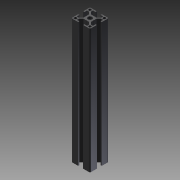
# Autodesk Inventor part: HFS6-3030-200
Saved by Autodesk Inventor 2011 SP1 (Build 150282100, 282)
## iProperties
Created: 2016-11-23
Part Number: HFS6-3030-200
Catalog Web Link: www.cadenas.de
Description: NEFS6-3030, NEFSB6-3030, EFS6-3030, EFSB6-3030, HFS6-3030, HFSB6-3030, CAF6-3030, HFSY6-3030, NFSL6-3030,  HFSL6-3030, HFSLB6-3030, GFS6-3030-HFS6 Series Aluminum Extrusions 30 Square -1 Slot-
Vendor: MISUMI
Document SubType Name: Modeling
Designer: psAdmin
Manufacturer: MISUMI
Mass: 66.3829 g
Surface Area: 634.997 cm^2
Volume: 66.3829 cm^3
Density: 1 g/cm^3
Category: PARTsolutions
Company: MISUMI
Title: HFS6-3030-200
Author: Cadenas PARTsolutions
Comments: HFS6 Series Aluminum Extrusions 30 Square -1 Slot-
PSOL_IDENT_0: {$CADENAS_DATA\23d-libs\misumi\metric\38_al_extrusions_blackets\6\hfs6_3030.prj},609 {VTYP=3D},{NB=H
PSOL_IDENT_1: FS6-3030-200},{LINA=HFS6-3030-200},{NN=NEFS6-3030, NEFSB6-3030, EFS6-3030, EFSB6-3030, HFS6-3030, HF
PSOL_IDENT_2: SB6-3030, CAF6-3030, HFSY6-3030, NFSL6-3030,  HFSL6-3030, HFSLB6-3030, GFS6-3030},{DATE=17.06.2016 0
PSOL_IDENT_3: 5:53:17},{GEOMDATE=28.10.2014 00:00:00},{VERSION=},{LINEID=130},{LINESUBID=-1},{WBVAR=L,ALT1,ALT2,AL
PSOL_IDENT_4: T3,ALT4,ALT5,CP5,DL5,DR5,ALT6,ALT9,ALT10,ALT11,DD6SE,DD6,HP6,NHL6,DL6,NHR6,DR6,ALT7,ALT8,NH9,AH,BH,C
PSOL_IDENT_5: H,DH,EH,NH10,AV,BV,CV,DV,EV,NH11,AP,BP,CP,DP,EP,ALT12,ALT13,Z,NH12,XA,XB,XC,XD,XE,NH13,YA,YB,YC,YD,Y
PSOL_IDENT_6: E,ALT14,HP14,DL14,DR14,ALT15,HP15,DL15,DR15,ALT16,HP16,DL16,DR16,ALT17,HQ17,JLP,ALT19,ALT20}  {NB=HF
PSOL_IDENT_7: S6-3030-200},{LINA=HFS6-3030-200},{KT=DUMMY},{PN=HFS6-3030-200},{TPS=HFS6-3030},{MAT=A6N01SS-T5 Alum
PSOL_IDENT_8: inum Alloy},{ST=Clear Anodize},{FRMW=30},{FRMH=30},{FRD=6.8},{L=200.0},{MASS=0.90},{SA=333},{LX=2.83
PSOL_IDENT_9: x10^4},{LY=2.83x10^4},{ALT1=},{M1=0},{IDM1=6.647},{DALT1=4.2},{DPL1=0},{DPR1=0},{ALT1PN=},{ALT2=},{A
PSOL_IDENT_10: LT2ALG= '','w/o End Tapping (Heli-Coil Insert)','LHP','with LHP (Tapping on the Left (Heli-Coil Inse
PSOL_IDENT_11: rt))','RHP','with RHP (Tapping on the Right (Heli-Coil Insert))','HPW','with HPW (Tapping on Both En
PSOL_IDENT_12: ds (Heli-Coil Insert))' },{M2=0},{DP2=0},{ALT2PN=},{ALT3=},{ALT3ALG= '','w/o Tapping (Corner Section
PSOL_IDENT_13: )','LSP','with LSP (Tapping (Corner Section))','RSP','with RSP (Tapping (Corner Section))','SPW','wi
PSOL_IDENT_14: th SPW (Tapping (Corner Section))' },{M3=0},{IDM3=4.134},{DP3=0},{ALT3PN=},{ALT4=},{ALT4ALG= '', 'w/
PSOL_IDENT_15: o SC (High Precision Cut)', 'SC', 'with SC (High Precision Cut)' },{ALT4PN=},{ALT5=},{ALT5ALG= '','w
PSOL_IDENT_16: /o 45 Degree Cut','1','with 45 Degree Cut' },{CP5=},{CP5ALG= '','N/A' },{DL5=},{DL5ALG= '','N/A' },{
PSOL_IDENT_17: DR5=},{DR5ALG= '','N/A' },{FRMLALT5=0},{FRMRALT5=0},{ALT5PN=},{ALT6=},{ALT6ALG= '','w/o Fastening Lo
PSOL_IDENT_18: cation Wrench Access Hole Alterations','1','with Fastening Location Wrench Access Hole Alterations'
PSOL_IDENT_19: },{ALT9=},{ALT9ALG= '','w/o Location Specified Wrench Access Hole Alteratons (Horizontal)','1','with
PSOL_IDENT_20: Location Specified Wrench Access Hole Alteratons (Horizontal)' },{ALT10=},{ALT10ALG= '','w/o Locati
PSOL_IDENT_21: on Specified Wrench Access Hole Alteratons (Vertical)','1','with Location Specified Wrench Access Ho
PSOL_IDENT_22: le Alteratons (Vertical)' },{ALT11=},{ALT11ALG= '','w/o Location Specified Wrench Access Hole Altera
PSOL_IDENT_23: tons (Crisscross)','1','with Location Specified Wrench Access Hole Alteratons (Crisscross)' },{DD6SE=
PSOL_IDENT_24: },{DD6SEALG= '','N/A' },{DD6=0},{DD6ALG=0},{HP6=},{HP6ALG= '','N/A' },{NHL6=},{NHL6ALG= '','N/A' },{
PSOL_IDENT_25: DL6=},{DL6ALG= '','N/A' },{NHR6=},{NHR6ALG= '','N/A' },{DR6=},{DR6ALG= '','N/A' },{DD6PN=},{HL6=0},{
PSOL_IDENT_26: HL6D=0},{HR6=0},{HR6D=0},{J6=0},{J6D=0},{K6=0},{K6D=0},{ALT7=},{ALT7ALG= '','N/A' },{ALT8=},{ALT8ALG=
PSOL_IDENT_27: '','N/A' },{ALT678PN=},{NH9=0},{NH9MAX=5},{NH9ALG=[0]},{AH=0.0},{AHMIN=7},{AHMAX=195},{AHALG=[0]},{
PSOL_IDENT_28: BH=0.0},{BHMIN=2},{BHMAX=197},{BHALG=[0]},{CH=0.0},{CHMIN=2},{CHMAX=199},{CHALG=[0]},{DH=0.0},{DHMIN=
PSOL_IDENT_29: 2},{DHMAX=201},{DHALG=[0]},{EH=0.0},{EHMIN=2},{EHMAX=193},{EHALG=[0]},{NH10=0},{NH10MAX=5},{NH10ALG=
PSOL_IDENT_30: [0]},{AV=0.0},{AVMIN=7},{AVMAX=195},{AVALG=[0]},{BV=0.0},{BVMIN=2},{BVMAX=197},{BVALG=[0]},{CV=0.0},
PSOL_IDENT_31: {CVMIN=2},{CVMAX=199},{CVALG=[0]},{DV=0.0},{DVMIN=2},{DVMAX=201},{DVALG=[0]},{EV=0.0},{EVMIN=2},{EVM
PSOL_IDENT_32: AX=193},{EVALG=[0]},{NH11=0},{NH11MAX=5},{NH11ALG=[0]},{AP=0.0},{APMIN=7},{APMAX=195},{APALG=[0]},{B
PSOL_IDENT_33: P=0.0},{BPMIN=2},{BPMAX=197},{BPALG=[0]},{CP=0.0},{CPMIN=2},{CPMAX=199},{CPALG=[0]},{DP=0.0},{DPMIN=
PSOL_IDENT_34: 2},{DPMAX=201},{DPALG=[0]},{EP=0.0},{EPMIN=2},{EPMAX=193},{EPALG=[0]},{ALT9PN=},{ALT10PN=},{ALT11PN=
PSOL_IDENT_35: },{ALT91011PN=},{ALT12=},{ALT12ALG= '','w/o Counterbore Hole in Specified Position (Vertical)','1','
PSOL_IDENT_36: with Counterbore Hole in Specified Position (Vertical)' },{ALT13=},{ALT13ALG= '','w/o Counterbore Ho
PSOL_IDENT_37: le in Specified Position (Horizontal)','1','with Counterbore Hole in Specified Position (Horizontal)'
PSOL_IDENT_38: },{Z=},{ZALG= '','N/A' },{DD12=0.0},{DD112=0.0},{NH12=0},{NH12MAX=5},{NH12ALG=[0]},{XA=0.0},{XAMIN=
PSOL_IDENT_39: 7},{XAMAX=195},{XAALG=[0]},{XB=0.0},{XBMIN=2},{XBMAX=197},{XBALG=[0]},{XC=0.0},{XCMIN=2},{XCMAX=199}
PSOL_IDENT_40: ,{XCALG=[0]},{XD=0.0},{XDMIN=2},{XDMAX=201},{XDALG=[0]},{XE=0.0},{XEMIN=2},{XEMAX=193},{XEALG=[0]},{
PSOL_IDENT_41: NH13=0},{NH13MAX=5},{NH13ALG=[0]},{YA=0.0},{YAMIN=7},{YAMAX=195},{YAALG=[0]},{YB=0.0},{YBMIN=2},{YBM
PSOL_IDENT_42: AX=197},{YBALG=[0]},{YC=0.0},{YCMIN=2},{YCMAX=199},{YCALG=[0]},{YD=0.0},{YDMIN=2},{YDMAX=201},{YDALG=
PSOL_IDENT_43: [0]},{YE=0.0},{YEMIN=2},{YEMAX=193},{YEALG=[0]},{ALT12PN=},{ALT13PN=},{ALT1213PN=},{ALT14=},{ALT14AL
PSOL_IDENT_44: G= '','w/o D Type Hole Alteration','1','with D Type Hole Alteration' },{HP14=},{HP14ALG= '','N/A' },
PSOL_IDENT_45: {DL14=},{DL14ALG= '','N/A' },{DR14=},{DR14ALG= '','N/A' },{H14=0},{D14=0.0},{ALT14PN=},{ALT15=},{ALT
PSOL_IDENT_46: 15ALG= '','w/o S Type Hole Alteration','1','with S Type Hole Alteration' },{HP15=},{HP15ALG= '','N/A'
PSOL_IDENT_47: },{DL15=},{DL15ALG= '','N/A' },{DR15=},{DR15ALG= '','N/A' },{H15=0},{D115=0.0},{D215=0.0},{ALT15PN=
PSOL_IDENT_48: },{ALT16=},{ALT16ALG= '','w/o M Type Hole Alteration','1','with M Type Hole Alteration' },{HP16=},{H
PSOL_IDENT_49: P16ALG= '','N/A' },{DL16=},{DL16ALG= '','N/A' },{DR16=},{DR16ALG= '','N/A' },{H116=0},{D16=0.0},{ALT
PSOL_IDENT_50: 16PN=},{ALT17=},{ALT17ALG= '','w/o L Type Hole Alteration (Top)','1','with L Type Hole Alteration (T
PSOL_IDENT_51: op)' },{HQ17=0},{HQ17ALG=0},{JLP=0},{JLPMIN=4.9},{JLPMAX=0},{JLPALG=[0]},{L17=0},{D17=0.0},{ALT17PN=
PSOL_IDENT_52: },{ALT19=},{ALT19ALG= '','N/A' },{M19=0},{DP19=0},{ALT19PN=},{ALT20=},{ALT20PN=},{ERRORALT01=OK},{ER
PSOL_IDENT_53: RORALT02=OK},{ERRORALT03=OK},{ERRORALT05=OK},{ERRORALT06091=OK},{ERRORALT06092=OK},{ERRORALT06093=OK
PSOL_IDENT_54: },{ERRORALT06094=OK},{ERRORALT06101=OK},{ERRORALT06102=OK},{ERRORALT06103=OK},{ERRORALT06104=OK},{ER
PSOL_IDENT_55: RORALT06111=OK},{ERRORALT06112=OK},{ERRORALT06113=OK},{ERRORALT06114=OK},{ERRORALT06121=OK},{ERRORAL
PSOL_IDENT_56: T06122=OK},{ERRORALT06123=OK},{ERRORALT06124=OK},{ERRORALT06131=OK},{ERRORALT06132=OK},{ERRORALT0613
PSOL_IDENT_57: 3=OK},{ERRORALT06134=OK},{ERRORALT0614=OK},{ERRORALT0615=OK},{ERRORALT0616=OK},{ERRORALT06171=OK},{E
PSOL_IDENT_58: RRORALT06172=OK},{ERRORALT06173=OK},{ERRORALT0619=OK},{ERRORALT0911=OK},{ERRORALT0913=OK},{ERRORALT0
PSOL_IDENT_59: 914=OK},{ERRORALT0915=OK},{ERRORALT0916=OK},{ERRORALT0917=OK},{ERRORALT0919=OK},{ERRORALT1011=OK},{E
PSOL_IDENT_60: RRORALT1012=OK},{ERRORALT1014=OK},{ERRORALT1015=OK},{ERRORALT1016=OK},{ERRORALT1017=OK},{ERRORALT101
PSOL_IDENT_61: 9=OK},{ERRORALT1112=OK},{ERRORALT1113=OK},{ERRORALT1114=OK},{ERRORALT1115=OK},{ERRORALT1116=OK},{ERR
PSOL_IDENT_62: ORALT1117=OK},{ERRORALT1119=OK},{ERRORALT1214=OK},{ERRORALT1215=OK},{ERRORALT1216=OK},{ERRORALT1217=
PSOL_IDENT_63: OK},{ERRORALT1219=OK},{ERRORALT1314=OK},{ERRORALT1315=OK},{ERRORALT1316=OK},{ERRORALT1317=OK},{ERROR
PSOL_IDENT_64: ALT1319=OK},{ERRORALT1415=OK},{ERRORALT1416=OK},{ERRORALT1417=OK},{ERRORALT1419=OK},{ERRORALT1516=OK
PSOL_IDENT_65: },{ERRORALT1517=OK},{ERRORALT1519=OK},{ERRORALT1617=OK},{ERRORALT1619=OK},{ERRORALT1719=OK},{ERRORPN=
PSOL_IDENT_66: }
NN: NEFS6-3030, NEFSB6-3030, EFS6-3030, EFSB6-3030, HFS6-3030, HFSB6-3030, CAF6-3030, HFSY6-3030, NFSL6-3030,  HFSL6-3030, HFSLB6-3030, GFS6-3030
NT: HFS6 Series Aluminum Extrusions 30 Square -1 Slot-
NB: HFS6-3030-200
NBSYN: $PN.
LINA: HFS6-3030-200
PN: HFS6-3030-200
TPS: HFS6-3030
MAT: A6N01SS-T5 Aluminum Alloy
ST: Clear Anodize
L: 200.0
MASS: 0.90
SA: 333
LX: 2.83x10^4
LY: 2.83x10^4
ALT1: w/o End Tapping
M1: 0
DPL1: 0
DPR1: 0
ALT2: w/o End Tapping (Heli-Coil Insert)
M2: 0
DP2: 0
ALT3: w/o Tapping (Corner Section)
M3: 0
DP3: 0
ALT4: w/o SC (High Precision Cut)
ALT5: w/o 45 Degree Cut
CP5: N/A
DL5: N/A
DR5: N/A
ALT6: w/o Fastening Location Wrench Access Hole Alterations
ALT9: w/o Location Specified Wrench Access Hole Alteratons (Horizontal)
ALT10: w/o Location Specified Wrench Access Hole Alteratons (Vertical)
ALT11: w/o Location Specified Wrench Access Hole Alteratons (Crisscross)
DD6SE: N/A
DD6: 0
HP6: N/A
NHL6: N/A
DL6: N/A
NHR6: N/A
DR6: N/A
HL6D: 0
HR6D: 0
J6D: 0
K6D: 0
ALT7: N/A
ALT8: N/A
NH9: 0
AH: 0.0
BH: 0.0
CH: 0.0
DH: 0.0
EH: 0.0
NH10: 0
AV: 0.0
BV: 0.0
CV: 0.0
DV: 0.0
EV: 0.0
NH11: 0
AP: 0.0
BP: 0.0
CP: 0.0
DP: 0.0
EP: 0.0
ALT12: w/o Counterbore Hole in Specified Position (Vertical)
ALT13: w/o Counterbore Hole in Specified Position (Horizontal)
Z: N/A
DD12: 0.0
DD112: 0.0
NH12: 0
XA: 0.0
XB: 0.0
XC: 0.0
XD: 0.0
XE: 0.0
NH13: 0
YA: 0.0
YB: 0.0
YC: 0.0
YD: 0.0
YE: 0.0
ALT14: w/o D Type Hole Alteration
HP14: N/A
DL14: N/A
DR14: N/A
H14: 0
D14: 0.0
ALT15: w/o S Type Hole Alteration
HP15: N/A
DL15: N/A
DR15: N/A
H15: 0
D115: 0.0
D215: 0.0
ALT16: w/o M Type Hole Alteration
HP16: N/A
DL16: N/A
DR16: N/A
H116: 0
D16: 0.0
ALT17: w/o L Type Hole Alteration (Top)
HQ17: 0
JLP: 0
D17: 0.0
ALT19: N/A
M19: 0
DP19: 0
ALT20: w/o CW (End Face C Chamfering)
SUPPLIER: MISUMI
ARTICLENO: HFS6-3030-200
BOMINFO: HFS6-3030-200
CREATOR: CADENAS GmbH
Autodesk Inventor part; units mm, degrees
sketch "Sketch_1" plane through (0, 0, 0) normal (0, 0, 1) x (1, 0, 0)
  line L0 (-15, 4) -> (-13, 4)
  line L1 (-13, 4) -> (-13, 8.25)
  line L2 (-13, 8.25) -> (-9.6642, 8.25)
  line L3 (-9.6642, 8.25) -> (-6, 4.5858)
  line L4 (-6, 4.5858) -> (-6, 0.5196)
  line L5 (-6, 0.5196) -> (-5.7, 0)
  line L6 (-5.7, 0) -> (-6, -0.5196)
  line L7 (-6, -0.5196) -> (-6, -4.5858)
  line L8 (-6, -4.5858) -> (-9.6642, -8.25)
  line L9 (-9.6642, -8.25) -> (-13, -8.25)
  line L10 (-13, -8.25) -> (-13, -4)
  line L11 (-13, -4) -> (-15, -4)
  line L12 (-15, -4) -> (-15, -13)
  arc A0 (-15, -13) -> (-13, -15) centre (-13, -13) ccw
  line L13 (-13, -15) -> (-4, -15)
  line L14 (-4, -15) -> (-4, -13)
  line L15 (-4, -13) -> (-8.25, -13)
  line L16 (-8.25, -13) -> (-8.25, -9.6642)
  line L17 (-8.25, -9.6642) -> (-4.5858, -6)
  line L18 (-4.5858, -6) -> (-0.5196, -6)
  line L19 (-0.5196, -6) -> (0, -5.7)
  line L20 (0, -5.7) -> (0.5196, -6)
  line L21 (0.5196, -6) -> (4.5858, -6)
  line L22 (4.5858, -6) -> (8.25, -9.6642)
  line L23 (8.25, -9.6642) -> (8.25, -13)
  line L24 (8.25, -13) -> (4, -13)
  line L25 (4, -13) -> (4, -15)
  line L26 (4, -15) -> (13, -15)
  arc A1 (13, -15) -> (15, -13) centre (13, -13) ccw
  line L27 (15, -13) -> (15, -4)
  line L28 (15, -4) -> (13, -4)
  line L29 (13, -4) -> (13, -8.25)
  line L30 (13, -8.25) -> (9.6642, -8.25)
  line L31 (9.6642, -8.25) -> (6, -4.5858)
  line L32 (6, -4.5858) -> (6, -0.5196)
  line L33 (6, -0.5196) -> (5.7, 0)
  line L34 (5.7, 0) -> (6, 0.5196)
  line L35 (6, 0.5196) -> (6, 4.5858)
  line L36 (6, 4.5858) -> (9.6642, 8.25)
  line L37 (9.6642, 8.25) -> (13, 8.25)
  line L38 (13, 8.25) -> (13, 4)
  line L39 (13, 4) -> (15, 4)
  line L40 (15, 4) -> (15, 13)
  arc A2 (15, 13) -> (13, 15) centre (13, 13) ccw
  line L41 (13, 15) -> (4, 15)
  line L42 (4, 15) -> (4, 13)
  line L43 (4, 13) -> (8.25, 13)
  line L44 (8.25, 13) -> (8.25, 9.6642)
  line L45 (8.25, 9.6642) -> (4.5858, 6)
  line L46 (4.5858, 6) -> (0.5196, 6)
  line L47 (0.5196, 6) -> (0, 5.7)
  line L48 (0, 5.7) -> (-0.5196, 6)
  line L49 (-0.5196, 6) -> (-4.5858, 6)
  line L50 (-4.5858, 6) -> (-8.25, 9.6642)
  line L51 (-8.25, 9.6642) -> (-8.25, 13)
  line L52 (-8.25, 13) -> (-4, 13)
  line L53 (-4, 13) -> (-4, 15)
  line L54 (-4, 15) -> (-13, 15)
  arc A3 (-13, 15) -> (-15, 13) centre (-13, 13) ccw
  line L55 (-15, 13) -> (-15, 4)
  constraints: 112 end point, 8 point on circle, 4 centre point
extrude "Extrusion1" add sketch "Sketch_1" against normal blind 200
sketch "Sketch2" plane through (0, 0, -200) normal (0, 0, -1) x (-1, 0, 0)
  point P0 (0, 0)
hole "Hole1" at (0, 0, -200) direction (0, 0, 1) diameter 6.8 depth 200
sketch "Sketch3" plane through (0, 0, -200) normal (0, 0, -1) x (-1, 0, 0)
  point P0 (-11.6, 11.6)
hole "Hole2" at (11.6, 11.6, -200) direction (0, 0, 1) diameter 4.2 depth 200
pattern_linear "Rectangular Pattern1" count 2 spacing 23.2 along (-1, 0, 0) count 2 spacing 23.2 along (0, -1, 0) of "Hole2"
ref_plane "C1_XY" through (0, 0, 0) normal (0, 0, 1) x (1, 0, 0)
ref_plane "C1_YZ" through (0, 0, 0) normal (1, 0, 0) x (0, 1, 0)
ref_plane "C1_ZX" through (0, 0, 0) normal (0, 1, 0) x (0, 0, 1)
ref_plane "to_frame_cap1_XY" through (0, 0, 0) normal (0, 0, 1) x (1, 0, 0)
ref_plane "to_frame_cap1_YZ" through (0, 0, 0) normal (1, 0, 0) x (0, 1, 0)
ref_plane "to_frame_cap1_ZX" through (0, 0, 0) normal (0, 1, 0) x (0, 0, 1)
ref_plane "to_frame_cap2_XY" through (0, 0, -200) normal (0, 0, -1) x (1, 0, 0)
ref_plane "to_frame_cap2_YZ" through (0, 0, -200) normal (1, 0, 0) x (0, -1, 0)
ref_plane "to_frame_cap2_ZX" through (0, 0, -200) normal (0, -1, 0) x (0, 0, -1)
body "Solid1"
